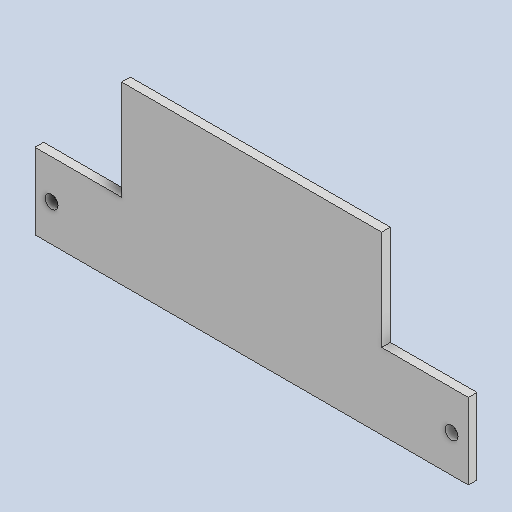
# Autodesk Inventor part: tylna
Saved by Autodesk Inventor 2023 (Build 270158000, 158)
## iProperties
Created: 2023-08-20
Part Number: tylna
Material: Ogólny
Document SubType Name: Modeling
Designer: Kamil
Density: 1 g/cm^3
Appearance: Domyślna
Author: Kamil
Autodesk Inventor part; units mm, degrees
ref_plane "YZ Plane" through (0, 0, 0) normal (1, 0, 0) x (0, 1, 0)
ref_plane "XZ Plane" through (0, 0, 0) normal (0, 1, 0) x (-1, 0, 0)
ref_plane "XY Plane" through (0, 0, 0) normal (0, 0, 1) x (1, 0, 0)
sketch "Szkic1" plane through (0, 0, 0) normal (0, 0, 1) x (1, 0, 0)
  line L0 (2.6774, 0.115) -> (-0.6, 0.115) projected
  spline S0 degree 3 poles (3.0833, -0.1968) (3.1541, -0.2257) (3.223, -0.256) (3.5835, -0.4251) (3.888, -0.6087) (4.4504, -1.0382) (4.7087, -1.2836) (5.1613, -1.7912) (5.3932, -2.1042) (5.7913, -2.77) (5.9577, -3.1227) (6.2121, -3.7972) (6.3223, -4.1828) (6.4663, -4.968) (6.5, -5.3675) (6.5, -5.7331) knots -1.428143 -1.428143 -1.428143 -1.428143 -1.406087 -1.406087 -1.308684 -1.308684 -1.211282 -1.211282 -1.104676 -1.104676 -0.99807 -0.99807 -0.888411 -0.888411 -0.778752 -0.778752 -0.778752 -0.778752 projected
  line L1 (6.5, -5.7331) -> (6.5, -13.1255) projected
  circle A0 centre (3.25, -5.9055) radius 1.5 projected
  line L2 (-0.6, 0) -> (-0.6, -13.1255) projected
  line L3 (-0.6, -13.4271) -> (99.4, -13.4271) projected
  line L4 (-0.6, -14.1019) -> (-0.6, -13.1255) projected
  line L5 (6.5, -14.1019) -> (6.5, -13.1255) projected
  line L6 (-0.6, -13.4271) -> (-0.6, -28.9827) projected
  line L7 (-0.6, -13.4271) -> (-0.6, -28.9827) projected
  line L8 (-0.6, -13.4271) -> (99.4, -13.4271)
  line L9 (99.4, -13.4271) -> (99.4, 3.0729)
  line L10 (99.4, 3.0729) -> (-0.6, 3.0729)
  line L11 (-0.6, 3.0729) -> (-0.6, -13.4271)
  point P0 (0, 0)
  dimension "d0" = 16.5
  constraints: 8 end point, 2 parallel, 1 horizontal, 1 perpendicular
  measures "d0" distance of L9.end L8.end
extrude "Wyciągnięcie proste1" add sketch "Szkic1" along normal blind 2 contours A0 | L11 L10 L9 L3 L4 L2
sketch "Szkic2" plane through (0, 0, 2) normal (0, 0, 1) x (1, 0, 0)
  line L0 (79.4, 9.1073) -> (19.4, 9.1073) projected
  line L1 (99.4, 3.0729) -> (-0.6, 3.0729) projected
  line L2 (79.4, 9.1073) -> (19.4, 9.1073)
  line L3 (19.4, 9.1073) -> (19.4, 3.0729)
  line L4 (19.4, 3.0729) -> (79.4, 3.0729)
  line L5 (79.4, 3.0729) -> (79.4, 9.1073)
  point P0 (0, 0)
  constraints: 8 end point, 2 parallel, 1 horizontal, 1 perpendicular, 1 point on line
extrude "Wyciągnięcie proste2" add sketch "Szkic2" against normal up to surface (2 mm away)
sketch "Szkic3" plane through (0, 0, 2) normal (0, 0, 1) x (1, 0, 0)
  line L0 (99.4, -13.4271) -> (99.4, 3.0729) projected
  line L1 (99.4, 3.0729) -> (79.4, 3.0729) projected
  line L2 (79.4, 3.0729) -> (79.4, 9.1073) projected
  line L3 (79.4, 9.1073) -> (19.4, 9.1073) projected
  line L4 (19.4, 9.1073) -> (19.4, 3.0729) projected
  line L5 (19.4, 3.0729) -> (-0.6, 3.0729) projected
  line L6 (-0.6, 3.0729) -> (-0.6, -13.4271) projected
  line L7 (-0.6, -13.4271) -> (99.4, -13.4271) projected
  line L8 (79.4, 9.1073) -> (19.4, 9.1073)
  line L9 (19.4, 9.1073) -> (19.4, 26.1073)
  line L10 (19.4, 26.1073) -> (79.4, 26.1073)
  line L11 (79.4, 26.1073) -> (79.4, 9.1073)
  point P0 (0, 0)
  dimension "d5" = 17
  constraints: 8 end point, 2 parallel, 1 horizontal, 1 perpendicular
  measures "d5" distance of L8.end L9.end
extrude "Wyciągnięcie proste3" add sketch "Szkic3" against normal blind 2 contours L3 L9 L10 L11
sketch "Szkic4" plane through (0, 0, 2) normal (0, 0, 1) x (1, 0, 0)
  circle A0 centre (3.25, -5.9055) radius 1.5 projected
  line L0 (79.4, 26.1073) -> (19.4, 26.1073) projected
  line L1 (19.4, 26.1073) -> (79.4, 26.1073) projected
  line L2 (49.4, 26.1073) -> (49.4, -13.4271)
  line L3 (-0.6, -13.4271) -> (99.4, -13.4271) projected
  circle A1 centre (95.55, -5.9055) radius 1.5
  point P0 (0, 0)
  constraints: 2 end point, 2 midpoint, 1 centre point, 1 symmetric about line, 1 other
extrude "Wyciągnięcie proste4" cut sketch "Szkic4" against normal through all
sketch "Szkic5" plane through (0, 0, 2) normal (0, 0, 1) x (1, 0, 0)
  line L0 (-0.6, -13.4271) -> (99.4, -13.4271) projected
  line L1 (-0.6, 3.0729) -> (-0.6, -13.4271) projected
  line L2 (-0.6, -13.4271) -> (99.4, -13.4271)
  line L3 (99.4, -13.4271) -> (99.4, -14.4271)
  line L4 (99.4, -14.4271) -> (-0.6, -14.4271)
  line L5 (-0.6, -14.4271) -> (-0.6, -13.4271)
  point P0 (0, 0)
  dimension "d10" = 1
  constraints: 8 end point, 2 parallel, 1 horizontal, 1 perpendicular
  measures "d10" distance of L2.end L3.end
extrude "Wyciągnięcie proste5" add sketch "Szkic5" against normal up to surface (2 mm away)
